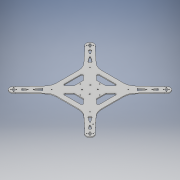
# Autodesk Inventor part: FirstLayer
Saved by Autodesk Inventor 2018 (Build 220112000, 112)
## iProperties
Created: 2019-09-30
Part Number: FirstLayer
Material: Generic
Document SubType Name: Modeling
Designer: anirudh
Density: 1 g/cm^3
Appearance: Default
Author: anirudh
Autodesk Inventor part; units mm, degrees
ref_plane "YZ Plane" through (0, 0, 0) normal (1, 0, 0) x (0, 1, 0)
ref_plane "XZ Plane" through (0, 0, 0) normal (0, 1, 0) x (-1, 0, 0)
ref_plane "XY Plane" through (0, 0, 0) normal (0, 0, 1) x (1, 0, 0)
sketch "Sketch1" plane through (0, 0, 0) normal (0, 1, 0) x (-1, 0, 0)
  line L0 (177.8, 0) -> (266.7, 0) construction
  circle A0 centre (240.6618, 62.8618) radius 5
  arc A1 (246.5851, 48.82) -> (226.62, 68.7851) centre (240.6618, 62.8618) ccw
  arc A2 (246.4085, 48.7468) -> (226.5468, 68.6085) centre (240.6618, 62.8618) ccw
  circle A3 centre (247.2379, 56.2857) radius 1.65
  circle A4 centre (247.2379, 56.2857) radius 1.65
  circle A5 centre (240.6618, 62.8618) radius 5
  circle A6 centre (246.1772, 68.3772) radius 1.65
  circle A7 centre (246.1772, 68.3772) radius 1.65
  circle A8 centre (234.0857, 69.4379) radius 1.65
  circle A9 centre (234.0857, 69.4379) radius 1.65
  circle A10 centre (235.1464, 57.3464) radius 1.65
  circle A11 centre (235.1464, 57.3464) radius 1.65
  arc A12 (226.7257, 42.3061) -> (226.983, 45.2157) centre (225.636, 43.8687) ccw
  arc A13 (226.7257, 42.3061) -> (226.983, 45.2157) centre (225.636, 43.8687) ccw
  arc A14 (223.0157, 49.183) -> (220.1061, 48.9257) centre (221.6687, 47.836) ccw
  arc A15 (223.0157, 49.183) -> (220.1061, 48.9257) centre (221.6687, 47.836) ccw
  arc A16 (210.9635, 35.8158) -> (213.6158, 33.1635) centre (212.5261, 34.7261) ccw
  arc A17 (210.9635, 35.8158) -> (213.6158, 33.1635) centre (212.5261, 34.7261) ccw
  line L1 (223.0157, 49.183) -> (226.983, 45.2157)
  line L2 (226.983, 45.2157) -> (223.0157, 49.183)
  line L3 (213.6158, 33.1635) -> (226.7257, 42.3061)
  line L4 (226.7257, 42.3061) -> (213.6158, 33.1635)
  line L5 (210.9635, 35.8158) -> (220.1061, 48.9257)
  line L6 (220.1061, 48.9257) -> (210.9635, 35.8158)
  arc A18 (213.6158, -210.9635) -> (210.9635, -213.6158) centre (212.5261, -212.5261) ccw
  arc A19 (213.6158, -210.9635) -> (210.9635, -213.6158) centre (212.5261, -212.5261) ccw
  line L7 (210.9635, -213.6158) -> (220.1061, -226.7257)
  line L8 (220.1061, -226.7257) -> (210.9635, -213.6158)
  line L9 (213.6158, -210.9635) -> (226.7257, -220.1061)
  line L10 (226.7257, -220.1061) -> (213.6158, -210.9635)
  arc A20 (226.983, -223.0157) -> (226.7257, -220.1061) centre (225.636, -221.6687) ccw
  arc A21 (226.983, -223.0157) -> (226.7257, -220.1061) centre (225.636, -221.6687) ccw
  line L11 (223.0157, -226.983) -> (226.983, -223.0157)
  line L12 (226.983, -223.0157) -> (223.0157, -226.983)
  circle A22 centre (235.1464, -235.1464) radius 1.65
  circle A23 centre (235.1464, -235.1464) radius 1.65
  circle A24 centre (240.6618, -240.6618) radius 5
  arc A25 (226.62, -246.5851) -> (246.5851, -226.62) centre (240.6618, -240.6618) ccw
  arc A26 (226.5468, -246.4085) -> (246.4085, -226.5468) centre (240.6618, -240.6618) ccw
  circle A27 centre (247.2379, -234.0857) radius 1.65
  circle A28 centre (247.2379, -234.0857) radius 1.65
  circle A29 centre (240.6618, -240.6618) radius 5
  circle A30 centre (246.1772, -246.1772) radius 1.65
  circle A31 centre (246.1772, -246.1772) radius 1.65
  circle A32 centre (234.0857, -247.2379) radius 1.65
  circle A33 centre (234.0857, -247.2379) radius 1.65
  arc A34 (220.1061, -226.7257) -> (223.0157, -226.983) centre (221.6687, -225.636) ccw
  arc A35 (220.1061, -226.7257) -> (223.0157, -226.983) centre (221.6687, -225.636) ccw
  arc A36 (-35.8158, 33.1635) -> (-33.1635, 35.8158) centre (-34.7261, 34.7261) ccw
  arc A37 (-35.8158, 33.1635) -> (-33.1635, 35.8158) centre (-34.7261, 34.7261) ccw
  line L13 (-33.1635, 35.8158) -> (-42.3061, 48.9257)
  line L14 (-42.3061, 48.9257) -> (-33.1635, 35.8158)
  line L15 (-35.8158, 33.1635) -> (-48.9257, 42.3061)
  line L16 (-48.9257, 42.3061) -> (-35.8158, 33.1635)
  arc A38 (-49.183, 45.2157) -> (-48.9257, 42.3061) centre (-47.836, 43.8687) ccw
  arc A39 (-49.183, 45.2157) -> (-48.9257, 42.3061) centre (-47.836, 43.8687) ccw
  line L17 (-45.2157, 49.183) -> (-49.183, 45.2157)
  line L18 (-49.183, 45.2157) -> (-45.2157, 49.183)
  circle A40 centre (-57.3464, 57.3464) radius 1.65
  circle A41 centre (-57.3464, 57.3464) radius 1.65
  circle A42 centre (-62.8121, 62.9315) radius 5
  arc A43 (-48.7656, 68.8437) -> (-68.7465, 48.8944) centre (-62.8121, 62.9315) ccw
  arc A44 (-48.6926, 68.667) -> (-68.5699, 48.821) centre (-62.8121, 62.9315) ccw
  circle A45 centre (-69.4379, 56.2857) radius 1.65
  circle A46 centre (-69.4379, 56.2857) radius 1.65
  circle A47 centre (-62.8121, 62.9315) radius 5
  circle A48 centre (-68.3772, 68.3772) radius 1.65
  circle A49 centre (-68.3772, 68.3772) radius 1.65
  circle A50 centre (-56.2857, 69.4379) radius 1.65
  circle A51 centre (-56.2857, 69.4379) radius 1.65
  arc A52 (-42.3061, 48.9257) -> (-45.2157, 49.183) centre (-43.8687, 47.836) ccw
  arc A53 (-42.3061, 48.9257) -> (-45.2157, 49.183) centre (-43.8687, 47.836) ccw
  arc A54 (-48.9257, -220.1061) -> (-49.183, -223.0157) centre (-47.836, -221.6687) ccw
  arc A55 (-48.9257, -220.1061) -> (-49.183, -223.0157) centre (-47.836, -221.6687) ccw
  line L19 (-45.2157, -226.983) -> (-49.183, -223.0157)
  line L20 (-49.183, -223.0157) -> (-45.2157, -226.983)
  arc A56 (-45.2157, -226.983) -> (-42.3061, -226.7257) centre (-43.8687, -225.636) ccw
  arc A57 (-45.2157, -226.983) -> (-42.3061, -226.7257) centre (-43.8687, -225.636) ccw
  line L21 (-35.8158, -210.9635) -> (-48.9257, -220.1061)
  line L22 (-48.9257, -220.1061) -> (-35.8158, -210.9635)
  line L23 (-42.3061, -226.7257) -> (-33.1635, -213.6158)
  arc A58 (-33.1635, -213.6158) -> (-35.8158, -210.9635) centre (-34.7261, -212.5261) ccw
  arc A59 (-33.1635, -213.6158) -> (-35.8158, -210.9635) centre (-34.7261, -212.5261) ccw
  line L24 (-33.1635, -213.6158) -> (-42.3061, -226.7257)
  circle A60 centre (-56.2857, -247.2379) radius 1.65
  circle A61 centre (-56.2857, -247.2379) radius 1.65
  circle A62 centre (-57.3464, -235.1464) radius 1.65
  circle A63 centre (-68.3772, -246.1772) radius 1.65
  circle A64 centre (-62.8618, -240.6618) radius 5
  circle A65 centre (-62.8618, -240.6618) radius 5
  circle A66 centre (-69.4379, -234.0857) radius 1.65
  circle A67 centre (-69.4379, -234.0857) radius 1.65
  arc A68 (-68.6085, -226.5468) -> (-48.7468, -246.4085) centre (-62.8618, -240.6618) ccw
  arc A69 (-68.7851, -226.62) -> (-48.82, -246.5851) centre (-62.8618, -240.6618) ccw
  circle A70 centre (-68.3772, -246.1772) radius 1.65
  circle A71 centre (-57.3464, -235.1464) radius 1.65
  line L25 (75.45, -106.9) -> (71.85, -106.9)
  line L26 (102.35, -104.15) -> (102.35, -106.9)
  line L27 (102.35, -106.9) -> (105.95, -106.9)
  line L28 (102.35, -70.9) -> (105.95, -70.9)
  line L29 (75.45, -73.65) -> (75.45, -70.9)
  line L30 (75.45, -70.9) -> (71.85, -70.9)
  arc A72 (71.85, -73.65) -> (75.45, -73.65) centre (73.65, -73.65) ccw
  line L31 (75.45, -73.65) -> (75.45, -70.9)
  line L32 (71.85, -70.9) -> (71.85, -73.65)
  arc A73 (71.85, -73.65) -> (75.45, -73.65) centre (73.65, -73.65) ccw
  arc A74 (75.45, -104.15) -> (71.85, -104.15) centre (73.65, -104.15) ccw
  arc A75 (75.45, -104.15) -> (71.85, -104.15) centre (73.65, -104.15) ccw
  arc A76 (105.95, -104.15) -> (102.35, -104.15) centre (104.15, -104.15) ccw
  arc A77 (105.95, -104.15) -> (102.35, -104.15) centre (104.15, -104.15) ccw
  arc A78 (102.35, -73.65) -> (105.95, -73.65) centre (104.15, -73.65) ccw
  arc A79 (102.35, -73.65) -> (105.95, -73.65) centre (104.15, -73.65) ccw
  line L33 (105.95, -73.65) -> (105.95, -70.9)
  line L34 (102.35, -73.65) -> (102.35, -70.9)
  line L35 (105.95, -106.9) -> (105.95, -104.15)
  line L36 (102.35, -104.15) -> (102.35, -106.9)
  line L37 (75.45, -106.9) -> (75.45, -104.15)
  line L38 (75.45, -104.15) -> (75.45, -106.9)
  line L39 (71.85, -104.15) -> (71.85, -106.9)
  line L40 (152.4, 0) -> (226.5468, 68.6085)
  line L41 (177.8, -25.4) -> (246.4085, 48.7468)
  line L42 (-48.6926, 68.667) -> (25.4, 0)
  line L43 (152.4, -177.8) -> (226.5468, -246.4085)
  line L44 (-68.5699, 48.821) -> (0, -25.4)
  line L45 (-68.6085, -226.5468) -> (0, -152.4)
  line L46 (-48.7468, -246.4085) -> (25.4, -177.8)
  line L47 (246.4085, -226.5468) -> (177.8, -152.4)
  line L48 (25.4, 0) -> (152.4, 0)
  line L49 (177.8, -25.4) -> (177.8, -152.4)
  line L50 (152.4, -177.8) -> (25.4, -177.8)
  line L51 (0, -25.4) -> (0, -152.4)
  arc A80 (202.4073, 21.9521) -> (199.7521, 24.6073) centre (200.8517, 23.0517) ccw
  arc A81 (202.4073, 21.9521) -> (199.7521, 24.6073) centre (200.8517, 23.0517) ccw
  arc A82 (180.0144, 10.6538) -> (179.767, 7.7512) centre (181.114, 9.0983) ccw
  arc A83 (180.0144, 10.6538) -> (179.767, 7.7512) centre (181.114, 9.0983) ccw
  arc A84 (185.5512, 1.967) -> (188.4538, 2.2144) centre (186.8983, 3.314) ccw
  arc A85 (185.5512, 1.967) -> (188.4538, 2.2144) centre (186.8983, 3.314) ccw
  line L52 (199.7521, 24.6073) -> (180.0144, 10.6538)
  line L53 (199.7521, 24.6073) -> (180.0144, 10.6538)
  line L54 (202.4073, 21.9521) -> (188.4538, 2.2144)
  line L55 (202.4073, 21.9521) -> (188.4538, 2.2144)
  line L56 (179.767, 7.7512) -> (185.5512, 1.967)
  line L57 (185.5512, 1.967) -> (179.767, 7.7512)
  arc A86 (199.7521, -202.4073) -> (202.4073, -199.7521) centre (200.8517, -200.8517) ccw
  arc A87 (199.7521, -202.4073) -> (202.4073, -199.7521) centre (200.8517, -200.8517) ccw
  arc A88 (179.767, -185.5512) -> (180.0144, -188.4538) centre (181.114, -186.8983) ccw
  arc A89 (188.4538, -180.0144) -> (185.5512, -179.767) centre (186.8983, -181.114) ccw
  arc A90 (188.4538, -180.0144) -> (185.5512, -179.767) centre (186.8983, -181.114) ccw
  line L58 (199.7521, -202.4073) -> (180.0144, -188.4538)
  line L59 (202.4073, -199.7521) -> (188.4538, -180.0144)
  line L60 (179.767, -185.5512) -> (185.5512, -179.767)
  arc A91 (-21.9521, 24.6073) -> (-24.6073, 21.9521) centre (-23.0517, 23.0517) ccw
  arc A92 (-1.967, 7.7512) -> (-2.2144, 10.6538) centre (-3.314, 9.0983) ccw
  arc A93 (-1.967, 7.7512) -> (-2.2144, 10.6538) centre (-3.314, 9.0983) ccw
  arc A94 (-10.6538, 2.2144) -> (-7.7512, 1.967) centre (-9.0983, 3.314) ccw
  arc A95 (-10.6538, 2.2144) -> (-7.7512, 1.967) centre (-9.0983, 3.314) ccw
  line L61 (-21.9521, 24.6073) -> (-2.2144, 10.6538)
  line L62 (-21.9521, 24.6073) -> (-2.2144, 10.6538)
  line L63 (-24.6073, 21.9521) -> (-10.6538, 2.2144)
  line L64 (-1.967, 7.7512) -> (-7.7512, 1.967)
  line L65 (-7.7512, 1.967) -> (-1.967, 7.7512)
  arc A96 (-24.6073, -199.7521) -> (-21.9521, -202.4073) centre (-23.0517, -200.8517) ccw
  line L66 (-21.9521, -202.4073) -> (-2.2144, -188.4538)
  line L67 (-24.6073, -199.7521) -> (-10.6538, -180.0144)
  arc A97 (-7.7512, -179.767) -> (-10.6538, -180.0144) centre (-9.0983, -181.114) ccw
  arc A98 (-2.2144, -188.4538) -> (-1.967, -185.5512) centre (-3.314, -186.8983) ccw
  line L68 (-1.967, -185.5512) -> (-7.7512, -179.767)
  circle A99 centre (12.7, -12.7) radius 1.75
  circle A100 centre (-36.9254, 24.525) radius 1.85
  circle A101 centre (12.7, -165.1) radius 1.75
  circle A102 centre (165.1, -12.7) radius 1.75
  circle A103 centre (165.1, -165.1) radius 1.75
  circle A104 centre (88.9, -50.8) radius 1.75
  circle A105 centre (127, -88.9) radius 1.75
  circle A106 centre (88.9, -127) radius 1.75
  circle A107 centre (50.8, -88.9) radius 1.75
  line L69 (88.9, -44.45) -> (107.95, -44.45)
  line L70 (107.95, -44.45) -> (69.85, -44.45)
  line L71 (88.9, -19.05) -> (133.35, -19.05)
  line L72 (133.35, -19.05) -> (44.45, -19.05)
  line L73 (44.45, -19.05) -> (69.85, -44.45)
  line L74 (107.95, -44.45) -> (133.35, -19.05)
  circle A108 centre (88.9, -127) radius 1.75
  line L75 (88.9, -133.35) -> (107.95, -133.35)
  line L76 (107.95, -133.35) -> (69.85, -133.35)
  line L77 (88.9, -158.75) -> (133.35, -158.75)
  line L78 (133.35, -158.75) -> (44.45, -158.75)
  line L79 (44.45, -158.75) -> (69.85, -133.35)
  line L80 (107.95, -133.35) -> (133.35, -158.75)
  line L81 (158.75, -88.9) -> (158.75, -44.45)
  line L82 (158.75, -44.45) -> (158.75, -133.35)
  line L83 (133.35, -88.9) -> (133.35, -69.85)
  line L84 (133.35, -69.85) -> (133.35, -107.95)
  line L85 (158.75, -44.45) -> (133.35, -69.85)
  line L86 (158.75, -133.35) -> (133.35, -107.95)
  line L87 (69.85, -44.45) -> (44.45, -19.05)
  line L88 (19.05, -88.9) -> (19.05, -44.45)
  line L89 (19.05, -44.45) -> (19.05, -133.35)
  line L90 (44.45, -88.9) -> (44.45, -69.85)
  line L91 (44.45, -69.85) -> (44.45, -107.95)
  line L92 (19.05, -44.45) -> (44.45, -69.85)
  line L93 (19.05, -133.35) -> (44.45, -107.95)
  point P0 (0, 0)
  point P1 (246.2412, 48.6311)
  point P2 (226.4311, 68.4412)
  point P3 (226.4311, -246.2412)
  point P4 (246.2412, -226.4311)
  point P5 (-88.9, 0)
  point P6 (-48.6311, 68.4412)
  point P7 (-68.4412, -226.4311)
  point P8 (-48.6311, -246.2412)
  point P9 (0, 0)
  constraints: 188 end point, 122 point on circle, 109 centre point, 45 coincident, 12 tangent, 8 equal length, 4 perpendicular, 4 vertical, 3 horizontal, 2 point on line, 1 concentric
extrude "Extrusion3" add sketch "Sketch1" along normal blind 3.175
fillet "Fillet4" radius 5.08 16 edges at (-44.45, 1.5875, -19.05) (-69.85, 1.5875, -44.45) (-107.95, 1.5875, -44.45) (-133.35, 1.5875, -19.05) (-19.05, 1.5875, -44.45) (-44.45, 1.5875, -69.85) (-44.45, 1.5875, -107.95) (-19.05, 1.5875, -133.35) (-44.45, 1.5875, -158.75) (-69.85, 1.5875, -133.35) (-107.95, 1.5875, -133.35) (-133.35, 1.5875, -158.75) (-158.75, 1.5875, -44.45) (-133.35, 1.5875, -69.85) (-133.35, 1.5875, -107.95) (-158.75, 1.5875, -133.35)
fillet "Fillet5" radius 50.8 8 edges at (-152.4, 1.5875, 0) (-25.4, 1.5875, 0) (0, 1.5875, -25.4) (-177.8, 1.5875, -25.4) (-177.8, 1.5875, -152.4) (-152.4, 1.5875, -177.8) (0, 1.5875, -152.4) (-25.4, 1.5875, -177.8)
body "Solid3"
